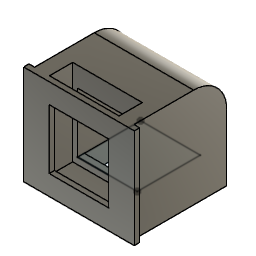
Fan Holder v4 (Autodesk Fusion 360 design; units mm, degrees)
Autodesk Fusion 360 part; units mm, degrees
sketch "Sketch1" plane through (0, 0, 0) normal (0, 0, 1) x (1, 0, 0)
  line L0 (0, 0) -> (-30, 0)
  line L1 (-30, 0) -> (-30, 30)
  line L2 (-30, 30) -> (0, 30)
  line L3 (0, 30) -> (0, 0)
  dimension "d1" = 30
  dimension "d2" = 30
  constraint horizontal L0
  constraint vertical L1
  constraint horizontal L2
  constraint vertical L3
  constraint coincident L0.start L3.end
  measures "d1" distance of L0.start L0.end
  measures "d2" distance of L0.start L2.end
extrude "Extrude1" add sketch "Sketch1" along normal blind 30
sketch "Sketch2" plane through (0, 0, 30) normal (0, 0, 1) x (-1, 0, 0)
  line L0 (0, -30) -> (30, -30)
  line L1 (30, -30) -> (30, 0)
  line L2 (30, 0) -> (0, 0)
  line L3 (0, 0) -> (0, -30)
  line L4 (30, 0) -> (25.5, 0)
  line L5 (25.5, 0) -> (25.5, -2)
  line L6 (25.5, -2) -> (30, -2)
  line L7 (30, -2) -> (30, 0)
  line L8 (25.5, -2) -> (4.5, -2)
  line L9 (4.5, -2) -> (4.5, -9)
  line L10 (4.5, -9) -> (25.5, -9)
  line L11 (25.5, -9) -> (25.5, -2)
  dimension "d5" = 4.5
  dimension "d6" = 2
  dimension "d7" = 21
  dimension "d8" = 7
  constraint horizontal L4
  constraint vertical L5
  constraint horizontal L6
  constraint vertical L7
  constraint coincident L1.end L2.start
  constraint horizontal L8
  constraint vertical L9
  constraint horizontal L10
  constraint vertical L11
  measures "d5" distance of L1.end L4.end
  measures "d6" distance of L1.end L6.end
  measures "d7" distance of L5.end L8.end
  measures "d8" distance of L5.end L10.end
extrude "Extrude2" cut sketch "Sketch2" against normal blind 25 contours L8 L9 L10 L11
sketch "Sketch3" plane through (0, 0, 0) normal (0, -1, 0) x (1, 0, 0)
  line L0 (-30, 0) -> (0, 0)
  line L1 (0, 0) -> (0, 30)
  line L2 (0, 30) -> (-30, 30)
  line L3 (-30, 30) -> (-30, 0)
  line L4 (-6, 6) -> (-24, 6)
  line L5 (-24, 6) -> (-24, 24)
  line L6 (-24, 24) -> (-6, 24)
  line L7 (-6, 24) -> (-6, 6)
  line L8 (-6, 6) -> (-24, 24) construction
  line L9 (-24, 6) -> (-6, 24) construction
  point P0 (-15, 15)
  dimension "d11" = 18
  dimension "d12" = 18
  constraint horizontal L4
  constraint perpendicular L4 L5
  constraint parallel L4 L6
  constraint parallel L5 L7
  constraint coincident L8 P0
  constraint coincident L9 P0
  measures "d11" distance of L5.end L6.end
  measures "d12" distance of L4.end L5.end
extrude "Extrude3" cut sketch "Sketch3" against normal blind 2 contours L4 L5 L6 L7
sketch "Sketch4" plane through (0, 0, 0) normal (1, 0, 0) x (0, 1, 0)
  line L0 (0, 0) -> (30, 0)
  line L1 (30, 0) -> (30, 30)
  line L2 (30, 30) -> (0, 30)
  line L3 (0, 30) -> (0, 0)
  line L4 (0, 0) -> (2, 0)
  line L5 (2, 0) -> (2, 30)
  line L6 (2, 30) -> (0, 30)
  line L7 (0, 30) -> (0, 0)
  dimension "d15" = 2
  dimension "d16" = 30
  constraint horizontal L4
  constraint vertical L5
  constraint horizontal L6
  constraint vertical L7
  constraint coincident L0.start L3.end
  measures "d15" distance of L0.start L4.end
  measures "d16" distance of L0.start L2.end
extrude "Extrude4" add sketch "Sketch4" along normal blind 2 contours L0 L2 L3 L4 L5 L6 L7
sketch "Sketch5" plane through (-30, 0, 0) normal (-1, 0, 0) x (0, -1, 0)
  line L0 (-30, 0) -> (0, 0)
  line L1 (0, 0) -> (0, 30)
  line L2 (0, 30) -> (-30, 30)
  line L3 (-30, 30) -> (-30, 0)
  line L4 (0, 0) -> (-2, 0)
  line L5 (-2, 0) -> (-2, 30)
  line L6 (-2, 30) -> (0, 30)
  line L7 (0, 30) -> (0, 0)
  dimension "d19" = 2
  dimension "d20" = 30
  constraint horizontal L4
  constraint vertical L5
  constraint horizontal L6
  constraint vertical L7
  constraint coincident L0.end L1.start
  measures "d19" distance of L0.end L4.end
  measures "d20" distance of L0.end L1.end
extrude "Extrude5" add sketch "Sketch5" along normal blind 2 contours L0 L1 L2 L4 L5 L6 L7
sketch "Sketch6" plane through (0, 0, 5) normal (0, 0, 1) x (-1, 0, 0)
  line L0 (25.5, -9) -> (25.5, -2)
  line L1 (25.5, -2) -> (4.5, -2)
  line L2 (4.5, -2) -> (4.5, -9)
  line L3 (4.5, -9) -> (25.5, -9)
  circle A0 centre (6, -5) radius 1
  dimension "d23" = 2
  measures "d23" diameter of A0
extrude "Extrude6" cut sketch "Sketch6" against normal blind 5 contours A0
sketch "Sketch7" plane through (0, 0, 0) normal (0, -1, 0) x (1, 0, 0)
  line L0 (-24, 6) -> (-24, 24)
  line L1 (-24, 24) -> (-6, 24)
  line L2 (-6, 24) -> (-6, 6)
  line L3 (-6, 6) -> (-24, 6)
  line L4 (-32, 0) -> (2, 0)
  line L5 (2, 0) -> (2, 30)
  line L6 (2, 30) -> (-32, 30)
  line L7 (-32, 30) -> (-32, 0)
  line L8 (-6, 6) -> (-24, 6)
  line L9 (-24, 6) -> (-24, 24)
  line L10 (-24, 24) -> (-6, 24)
  line L11 (-6, 24) -> (-6, 6)
  constraint horizontal L8
  constraint vertical L9
  constraint horizontal L10
  constraint vertical L11
  constraint coincident L0.end L1.start
  constraint coincident L2.end L3.start
extrude "Extrude7" cut sketch "Sketch7" against normal blind 28 contours L0 L1 L2 L3 L8 L9 L10 L11
fillet "Fillet1" radius 10 1 edges at (-15, 30, 30)
sketch "Sketch8" plane through (0, 0, 6) normal (0, 0, 1) x (-1, 0, 0)
  line L0 (24, -9) -> (6, -9)
  line L1 (6, -9) -> (6, -28)
  line L2 (6, -28) -> (24, -28)
  line L3 (24, -28) -> (24, -9)
  line L4 (24, -28) -> (6, -28)
  line L5 (6, -28) -> (6, -9)
  line L6 (6, -9) -> (24, -9)
  line L7 (24, -9) -> (24, -28)
  constraint horizontal L4
  constraint vertical L5
  constraint horizontal L6
  constraint vertical L7
  constraint coincident L0.end L1.start
  constraint coincident L2.end L3.start
sketch "Sketch9" plane through (0, 0, 6) normal (0, 0, 1) x (-1, 0, 0)
  line L0 (6, -9) -> (8, -9)
  line L1 (8, -9) -> (8, -11)
  line L2 (8, -11) -> (6, -11)
  line L3 (6, -11) -> (6, -9)
  line L4 (6, -11) -> (24, -11)
  line L5 (24, -11) -> (24, -28)
  line L6 (24, -28) -> (6, -28)
  line L7 (6, -28) -> (6, -11)
  point P0 (6, -9)
  point P1 (24, -28)
  dimension "d30" = 2
  dimension "d31" = 2
  constraint horizontal L0
  constraint vertical L1
  constraint horizontal L2
  constraint vertical L3
  constraint coincident P0 L0.start
  constraint horizontal L4
  constraint vertical L5
  constraint horizontal L6
  constraint vertical L7
  constraint coincident P1 L5.end
  measures "d30" distance of P0 L0.end
  measures "d31" distance of P0 L2.end
extrude "Extrude8" cut sketch "Sketch9" against normal blind 10 contours L2 L4 L5 L6 L7
extrude "Extrude9" cut 1 faces at (-29.3333, 0, 18) along direction (0, 1, 0) blind 0.2
sketch "Sketch10" plane through (0, 0, 0) normal (0, 0, -1) x (1, 0, 0)
  line L0 (2, -0.2) -> (-32, -0.2)
  line L1 (-32, -0.2) -> (-32, -2)
  line L2 (-32, -2) -> (-30, -2)
  line L3 (-30, -2) -> (-30, -30)
  line L4 (-30, -30) -> (0, -30)
  line L5 (0, -30) -> (0, -2)
  line L6 (0, -2) -> (2, -2)
  line L7 (2, -2) -> (2, -0.2)
  circle A0 centre (-6, -5) radius 1
  line L8 (-24, -28) -> (-24, -11)
  line L9 (-24, -11) -> (-6, -11)
  line L10 (-6, -11) -> (-6, -28)
  line L11 (-6, -28) -> (-24, -28)
extrude "Extrude10" add sketch "Sketch10" against normal blind 5 contours A0
extrude "Extrude11" cut 1 faces at (-11.5, 6.6667, 5) along direction (0, 0, -1) blind 1
sketch "Sketch11" plane through (0, 0, 4) normal (0, 0, 1) x (-1, 0, 0)
  line L0 (25.5, -9) -> (25.5, -2)
  line L1 (25.5, -2) -> (4.5, -2)
  line L2 (4.5, -2) -> (4.5, -9)
  line L3 (4.5, -9) -> (25.5, -9)
  circle A0 centre (8.1497, -5.5) radius 2
  dimension "d40" = 4
  measures "d40" diameter of A0
extrude "Extrude12" cut sketch "Sketch11" against normal blind 4 contours A0
extrude "Extrude13" cut 1 faces at (2, 0.8, 20) along direction (-1, 0, 0) blind 0.2
extrude "Extrude14" cut 1 faces at (-32, 1.4, 20) along direction (1, 0, 0) blind 0.2
extrude "Extrude15" cut 1 faces at (1.8, 0.8, 20) along direction (-1, 0, 0) blind 0.1
extrude "Extrude16" cut 1 faces at (-29.2, 0.2, 18) along direction (0, 1, 0) blind 0.2
extrude "Extrude17" cut 1 faces at (-31.8, 1.4667, 20) along direction (1, 0, 0) blind 0.1
